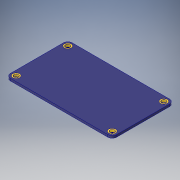
# Autodesk Inventor part: NX3224T024_011_PCB
Saved by Autodesk Inventor 2017 SP1 (Build 210196100, 196)
## iProperties
Created: 2016-08-28
Part Number: NX3224T024_011_PCB
Material: ABS Plastic
Document SubType Name: Modeling
Designer: jwrjc
Density: 1.06 g/cm^3
Appearance: Smooth - White
Author: jwrjc
Autodesk Inventor part; units mm, degrees
ref_plane "YZ Plane" through (0, 0, 0) normal (1, 0, 0) x (0, 1, 0)
ref_plane "XZ Plane" through (0, 0, 0) normal (0, 1, 0) x (-1, 0, 0)
ref_plane "XY Plane" through (0, 0, 0) normal (0, 0, 1) x (1, 0, 0)
sketch "Sketch1" plane through (0, 0, 0) normal (0, 1, 0) x (-1, 0, 0)
  line L0 (7.2999, 16.1677) -> (-29.7001, 16.1677)
  line L1 (-32.7001, 13.1677) -> (-32.7001, -54.8323)
  line L2 (-29.7001, -57.8323) -> (7.2999, -57.8323)
  line L3 (10.2999, -54.8323) -> (10.2999, 13.1677)
  circle A0 centre (6.7999, 12.6677) radius 1.6
  circle A1 centre (-29.2001, 12.6677) radius 1.6
  circle A2 centre (-29.2001, -54.3323) radius 1.6
  circle A3 centre (6.7999, -54.3323) radius 1.6
  arc A4 (10.2999, 13.1677) -> (7.2999, 16.1677) centre (7.2999, 13.1677) ccw
  arc A5 (-29.7001, 16.1677) -> (-32.7001, 13.1677) centre (-29.7001, 13.1677) ccw
  arc A6 (-32.7001, -54.8323) -> (-29.7001, -57.8323) centre (-29.7001, -54.8323) ccw
  arc A7 (7.2999, -57.8323) -> (10.2999, -54.8323) centre (7.2999, -54.8323) ccw
  point P0 (0, 0)
  point P1 (-32.7001, -57.8323)
  point P2 (-32.7001, 16.1677)
  point P3 (10.2999, -57.8323)
  dimension "d0" = 43
  dimension "d1" = 74
  dimension "d6" = 3.2
  dimension "d7" = 3.2
  dimension "d8" = 3.2
  dimension "d9" = 3.2
  dimension "d10" = 3
  dimension "d33" = 67
  dimension "d34" = 36
  dimension "d35" = 36
  constraints: 8 centre point, 8 end point, 8 point on circle, 8 tangent, 6 point on line, 3 equal radius, 2 parallel, 1 horizontal, 1 perpendicular
  measures "d0" distance of point (10.3, -57.832) point (-32.7, -57.832)
  measures "d1" distance of point (-32.7, -57.832) point (-32.7, 16.168)
  measures "d6" diameter of A0
  measures "d7" diameter of A1
  measures "d8" diameter of A2
  measures "d9" diameter of A3
  measures "d10" radius of A4
  measures "d33" distance of A2.centre A1.centre
  measures "d34" distance of A0.centre A1.centre
  measures "d35" distance of A3.centre A2.centre
extrude "Extrusion1" add sketch "Sketch1" along normal blind 1.6
sketch "Sketch2" plane through (0, 0, 0) normal (0, -1, 0) x (1, 0, 0)
  line L0 (32.7001, -54.8323) -> (32.7001, 13.1677) projected
  line L1 (29.7001, 16.1677) -> (-7.2999, 16.1677) projected
  line L2 (-7.2999, -57.8323) -> (29.7001, -57.8323) projected
  line L3 (32.7001, 16.1677) -> (32.7001, -57.8323) construction
  line L4 (32.7001, -57.8323) -> (-10.3024, -57.8323) construction
  line L5 (-10.3024, -57.8323) -> (-10.3024, 16.1677) construction
  line L6 (-10.3024, 16.1677) -> (32.7001, 16.1677) construction
  point P0 (0, 0)
  constraints: 3 collinear, 2 other
decal "Decal2"
sketch "Sketch3" plane through (0, 0, 0) normal (0, -1, 0) x (1, 0, 0)
  circle A0 centre (29.2001, 12.6677) radius 1.6 projected
  circle A1 centre (29.2001, 12.6677) radius 2.4
  circle A2 centre (-6.7999, 12.6677) radius 1.6 projected
  circle A3 centre (-6.7999, 12.6677) radius 2.4
  circle A4 centre (-6.7999, -54.3323) radius 1.6 projected
  circle A5 centre (-6.7999, -54.3323) radius 2.4
  circle A6 centre (29.2001, -54.3323) radius 2.4
  circle A7 centre (29.2001, 12.6677) radius 1.5
  circle A8 centre (-6.7999, 12.6677) radius 1.5
  circle A9 centre (-6.7999, -54.3323) radius 1.5
  circle A10 centre (29.2001, -54.3323) radius 1.5
  point P0 (0, 0)
  dimension "d57" = 4.8
  dimension "d58" = 4.8
  dimension "d59" = 4.8
  dimension "d60" = 4.8
  dimension "d61" = 3
  dimension "d62" = 3
  dimension "d63" = 3
  dimension "d64" = 3
  constraints: 8 centre point, 7 coincident
  measures "d57" diameter of A1
  measures "d58" diameter of A3
  measures "d59" diameter of A5
  measures "d60" diameter of A6
  measures "d61" diameter of A7
  measures "d62" diameter of A8
  measures "d63" diameter of A9
  measures "d64" diameter of A10
extrude "Extrusion2" add sketch "Sketch3" along normal blind 0.1 and the other way blind 1.7 separate body contours A0 | A1 | A2 | A3 | A4 | A5 | A6
body "Solid1"
body "Solid2"
